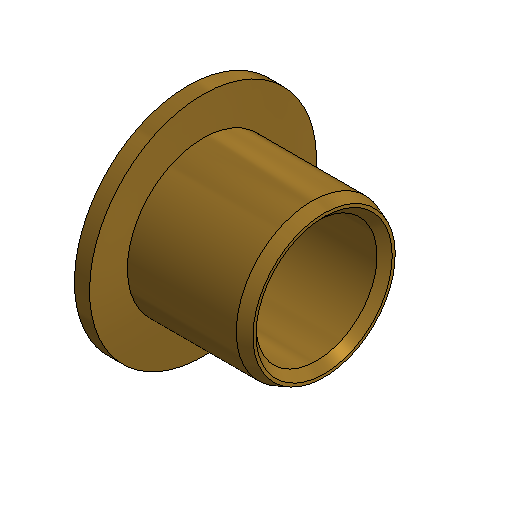
# Autodesk Inventor part: DU BUSH
Saved by Autodesk Inventor 2022.5 (Build 265521000, 521)
## iProperties
RuleStatus: InUse
Part Number: DU BUSH
Material: BC
Description: 3
Document SubType Name: Modeling
Designer: USER106
Density: 8.47 g/cm^3
Appearance: TIN Coating
MAKER: LUBO
Detail Description: Purchased products
Title: MB0808-15FDU
Author: USER106
Revision Number: D
Autodesk Inventor part; units mm, degrees
ref_plane "YZ Plane" through (0, 0, 0) normal (1, 0, 0) x (0, 1, 0)
ref_plane "XZ Plane" through (0, 0, 0) normal (0, 1, 0) x (-1, 0, 0)
ref_plane "XY Plane" through (0, 0, 0) normal (0, 0, 1) x (1, 0, 0)
sketch "Sketch2" plane through (0, 0, 0) normal (0, 1, 0) x (-1, 0, 0)
  line L0 (4.5, 4) -> (-4.5, 4)
  line L1 (4.5, 4) -> (4.5, 7.5)
  line L2 (4.5, 7.5) -> (3.5, 7.5)
  line L3 (3.5, 7.5) -> (3.5, 5)
  line L4 (3.5, 5) -> (-4.5, 5)
  line L5 (-4.5, 5) -> (-4.5, 4)
  line L6 (4.5, 0) -> (-4.5, 0)
  point P0 (0, 0)
  point P1 (0, 0)
  dimension "d1" = 9
  dimension "d2" = 1
  dimension "d3" = 1
  dimension "d4" = 3.5
  dimension "d5" = 8
  constraints: 14 end point, 4 perpendicular, 2 horizontal, 2 vertical alignment, 1 coincident, 1 midpoint, 1 vertical, 1 other
  measures "d1" distance of L0.start L0.end
  measures "d2" distance between parallel lines of L4 L0
  measures "d3" distance between parallel lines of L1 L3
  measures "d4" distance between parallel lines of L2 L0
  measures "d5" diameter of L0 L6
revolve "Revolution1" add sketch "Sketch2" angle 360 about axis through (-4.5, 0, 0) along (1, 0, 0)
fillet "Fillet1" radius 1 1 edges at (-4.5, 0, -4)
chamfer "Chamfer1" distance 0.5 angle 45 1 edges at (4.5, 0, -4)
chamfer "Chamfer2" distance 0.8 distance2 0.3 1 edges at (4.5, 0, -5) measured on face at (1.8333, 0.8021, 4.9353)
equation "\"d3\" = d2"
body "Solid1"
